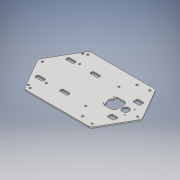
# Autodesk Inventor part: フレームC
Saved by Autodesk Inventor 2017 (Build 210142000, 142)
## iProperties
Created: 2016-08-20
Part Number: フレームC
Material: 一般
Document SubType Name: Modeling
Designer: NN
Density: 1 g/cm^3
Appearance: 既定
Mass: 23.9982 g
Surface Area: 257.222 cm^2
Volume: 23.9982 cm^3
Author: NN
Autodesk Inventor part; units mm, degrees
ref_plane "YZ Plane" through (0, 0, 0) normal (1, 0, 0) x (0, 1, 0)
ref_plane "XZ Plane" through (0, 0, 0) normal (0, 1, 0) x (-1, 0, 0)
ref_plane "XY Plane" through (0, 0, 0) normal (0, 0, 1) x (1, 0, 0)
sketch "スケッチ1" plane through (0, 0, 0) normal (0, 0, 1) x (1, 0, 0)
  line L0 (28.8675, 50) -> (57.735, 0)
  line L1 (57.735, 0) -> (28.8675, -50)
  line L2 (28.8675, -50) -> (-28.8675, -50)
  line L3 (-28.8675, -50) -> (-57.735, 0)
  line L4 (-57.735, 0) -> (-28.8675, 50)
  line L5 (-28.8675, 50) -> (28.8675, 50)
  point P0 (0, 0)
  point P1 (0, 0)
  dimension "d0" = 100
  constraints: 12 end point, 1 coincident, 1 horizontal, 13 other
  measures "d0" distance between parallel lines of L2 L5
extrude "押し出し1" add sketch "スケッチ1" along normal blind 2
sketch "スケッチ2" plane through (0, 0, 2) normal (0, 0, 1) x (1, 0, 0)
  line L0 (57.735, 0) -> (28.8675, 50) projected
  line L1 (28.8675, 50) -> (-28.8675, 50) projected
  line L2 (-28.8675, 50) -> (-57.735, 0) projected
  line L3 (-57.735, 0) -> (-28.8675, -50) projected
  line L4 (-28.8675, -50) -> (28.8675, -50) projected
  line L5 (28.8675, -50) -> (57.735, 0) projected
  line L6 (-50, 86.6025) -> (50, 86.6025)
  line L7 (50, 86.6025) -> (100, 0)
  line L8 (100, 0) -> (50, -86.6025)
  line L9 (50, -86.6025) -> (-50, -86.6025)
  line L10 (-50, -86.6025) -> (-100, 0)
  line L11 (-100, 0) -> (-50, 86.6025)
  line L12 (-28.8675, 50) -> (-71.1325, 50)
  line L13 (-28.8675, -50) -> (-71.1325, -50)
  point P0 (0, 0)
  dimension "d46" = 100
  constraints: 16 end point, 2 point on line, 1 horizontal, 1 parallel, 5 other
  measures "d46" distance of point (0, 0) L10.end
extrude "押し出し2" add sketch "スケッチ2" against normal up to surface (2 mm away) contours L2 L3 L13 L10 L11 L12
fillet "フィレット1" radius 7.5 6 edges at (-100, 0, 1) (-71.1325, -50, 1) (28.8675, -50, 1) (57.735, 0, 1) (28.8675, 50, 1) (-71.1325, 50, 1)
sketch "スケッチ3" plane through (0, 0, 0) normal (0, 0, -1) x (-1, 0, 0)
  arc A0 (73.2976, 46.25) -> (66.8024, 50) centre (66.8024, 42.5) ccw projected
  line L0 (66.8024, 50) -> (-24.5374, 50) projected
  arc A1 (-24.5374, 50) -> (-31.0326, 46.25) centre (-24.5374, 42.5) ccw projected
  line L1 (-31.0326, 46.25) -> (-55.57, 3.75) projected
  arc A2 (-55.57, 3.75) -> (-55.57, -3.75) centre (-49.0748, 0) ccw projected
  line L2 (-55.57, -3.75) -> (-31.0326, -46.25) projected
  arc A3 (-31.0326, -46.25) -> (-24.5374, -50) centre (-24.5374, -42.5) ccw projected
  line L3 (-24.5374, -50) -> (66.8024, -50) projected
  arc A4 (66.8024, -50) -> (73.2976, -46.25) centre (66.8024, -42.5) ccw projected
  line L4 (73.2976, -46.25) -> (97.8349, -3.75) projected
  arc A5 (97.8349, -3.75) -> (97.8349, 3.75) centre (91.3397, 0) ccw projected
  line L5 (97.8349, 3.75) -> (73.2976, 46.25) projected
  point P0 (0, 0)
hole "穴1" at (24.5374, -42.5, 0) at (49.0748, 0, 0) at (24.5374, 42.5, 0) at (-66.8024, 42.5, 0) at (-91.3397, 0, 0) at (-66.8024, -42.5, 0) direction (0, 0, 1) diameter 3 end through all
sketch "スケッチ4" plane through (0, 0, 2) normal (0, 0, 1) x (1, 0, 0)
  line L0 (-60.9252, 24.5) -> (-2.9252, 24.5)
  line L1 (-2.9252, 24.5) -> (-2.9252, -24.5)
  line L2 (-2.9252, -24.5) -> (-60.9252, -24.5)
  line L3 (-60.9252, -24.5) -> (-60.9252, 24.5)
  line L4 (-2.9252, 0) -> (0, 0)
  circle A0 centre (49.0748, 0) radius 1.5 projected
  dimension "d14" = 49
  dimension "d15" = 58
  dimension "d47" = 52
  constraints: 10 end point, 2 parallel, 2 perpendicular, 1 horizontal, 1 midpoint
  measures "d14" distance of L2.end L0.start
  measures "d15" distance of L0.start L0.end
  measures "d47" distance from line of A0.centre L1
hole "穴2" at (-2.9252, 24.5, 2) at (-2.9252, -24.5, 2) at (-60.9252, -24.5, 2) at (-60.9252, 24.5, 2) direction (0, 0, -1) diameter 2.7 end through all
sketch "スケッチ7" plane through (0, 0, 0) normal (0, 0, -1) x (-1, 0, 0)
  circle A0 centre (91.3397, 0) radius 1.5 projected
  line L0 (91.3397, 0) -> (41.7494, 0)
  line L1 (29.9252, -25) -> (41.9252, -25)
  line L2 (41.9252, -25) -> (41.9252, -20)
  line L3 (41.9252, -20) -> (29.9252, -20)
  line L4 (29.9252, -20) -> (29.9252, -25)
  line L5 (29.9252, 25) -> (41.9252, 25)
  line L6 (41.9252, 25) -> (41.9252, 20)
  line L7 (41.9252, 20) -> (29.9252, 20)
  line L8 (29.9252, 20) -> (29.9252, 25)
  circle A1 centre (60.9252, -24.5) radius 1.35 projected
  circle A2 centre (2.9252, 24.5) radius 1.35 projected
  circle A3 centre (2.9252, -24.5) radius 1.35 projected
  circle A4 centre (60.9252, 24.5) radius 1.35 projected
  circle A5 centre (91.3397, 0) radius 1.5 projected
  circle A6 centre (-24.5374, 42.5) radius 1.5 projected
  circle A7 centre (-24.5374, -42.5) radius 1.5 projected
  circle A8 centre (-49.0748, 0) radius 1.5 projected
  circle A9 centre (66.8024, 42.5) radius 1.5 projected
  circle A10 centre (66.8024, -42.5) radius 1.5 projected
  arc A11 (73.2976, 46.25) -> (66.8024, 50) centre (66.8024, 42.5) ccw projected
  line L9 (66.8024, 50) -> (-24.5374, 50) projected
  arc A12 (-24.5374, 50) -> (-31.0326, 46.25) centre (-24.5374, 42.5) ccw projected
  line L10 (-31.0326, 46.25) -> (-55.57, 3.75) projected
  arc A13 (-55.57, 3.75) -> (-55.57, -3.75) centre (-49.0748, 0) ccw projected
  line L11 (-55.57, -3.75) -> (-31.0326, -46.25) projected
  arc A14 (-31.0326, -46.25) -> (-24.5374, -50) centre (-24.5374, -42.5) ccw projected
  line L12 (-24.5374, -50) -> (66.8024, -50) projected
  arc A15 (66.8024, -50) -> (73.2976, -46.25) centre (66.8024, -42.5) ccw projected
  line L13 (73.2976, -46.25) -> (97.8349, -3.75) projected
  arc A16 (97.8349, -3.75) -> (97.8349, 3.75) centre (91.3397, 0) ccw projected
  line L14 (97.8349, 3.75) -> (73.2976, 46.25) projected
  point P0 (0, 0)
  dimension "d35" = 5
  dimension "d36" = 40
  dimension "d37" = 12
  dimension "d75" = 31
  constraints: 18 end point, 4 symmetric about line, 2 horizontal, 2 parallel, 1 perpendicular
  measures "d35" distance between parallel lines of L1 L3
  measures "d36" distance between parallel lines of L7 L3
  measures "d37" distance of L1.start L1.end
  measures "d75" distance from line of A1.centre L4
extrude "押し出し4" cut sketch "スケッチ7" against normal through all contours L4 L3 L2 L1 | L5 L6 L7 L8
fillet "フィレット2" radius 1.5 8 edges at (-41.9252, -25, 1) (-41.9252, -20, 1) (-29.9252, -25, 1) (-29.9252, -20, 1) (-41.9252, 20, 1) (-41.9252, 25, 1) (-29.9252, 20, 1) (-29.9252, 25, 1)
sketch "スケッチ9" plane through (0, 0, 2) normal (0, 0, 1) x (1, 0, 0)
  circle A0 centre (31.2748, 0.0001) radius 2.9 projected
  line L0 (17.0747, -8.7998) -> (17.0748, 8.8002) projected
  arc A1 (17.0748, 8.8002) -> (16.0748, 9.8002) centre (16.0748, 8.8002) ccw projected
  line L1 (16.0748, 9.8002) -> (9.5548, 9.8002) projected
  line L2 (8.5548, 5.1237) -> (8.5548, 8.8002) projected
  arc A2 (9.5548, 9.8002) -> (8.5548, 8.8002) centre (9.5548, 8.8002) ccw projected
  arc A3 (8.5548, 5.1237) -> (8.5547, -5.1233) centre (12.5548, 0.0002) ccw projected
  line L3 (8.5547, -8.7998) -> (8.5547, -5.1233) projected
  arc A4 (8.5547, -8.7998) -> (8.8406, -9.4998) centre (9.5547, -8.7998) ccw projected
  line L4 (16.0747, -9.7998) -> (9.5547, -9.7998) projected
  arc A5 (8.5547, -8.7998) -> (9.5547, -9.7998) centre (9.5547, -8.7998) ccw projected
  arc A6 (16.0747, -9.7998) -> (17.0747, -8.7998) centre (16.0747, -8.7998) ccw projected
  line L5 (17.1748, 8.8002) -> (17.1747, -8.7998)
  arc A7 (16.0747, -9.8998) -> (17.1747, -8.7998) centre (16.0747, -8.7998) ccw
  line L6 (16.0747, -9.8998) -> (9.5547, -9.8998)
  arc A8 (8.4547, -8.7998) -> (9.5547, -9.8998) centre (9.5547, -8.7998) ccw
  line L7 (8.4547, -8.7998) -> (8.4547, -5.1718)
  arc A9 (8.4548, 5.1722) -> (8.4547, -5.1718) centre (12.5548, 0.0002) ccw
  line L8 (8.4548, 5.1722) -> (8.4548, 8.8002)
  arc A10 (9.5548, 9.9002) -> (8.4548, 8.8002) centre (9.5548, 8.8002) ccw
  line L9 (9.5548, 9.9002) -> (16.0748, 9.9002)
  arc A11 (17.1748, 8.8002) -> (16.0748, 9.9002) centre (16.0748, 8.8002) ccw
  circle A12 centre (31.2748, 0.0001) radius 5
  point P0 (0, 0)
  dimension "d48" = 0.1
  dimension "d49" = 10
  constraints: 10 end point, 10 point on circle, 6 centre point, 1 coincident, 9 other
  measures "d48" distance between parallel lines of L5 L0
  measures "d49" diameter of A12
extrude "押し出し6" cut sketch "スケッチ9" against normal through all contours A0 | A6 L4 A5 A4 L3 A3 L2 A2 L1 A1 L0 | L5 A7 L6 A8 L7 A9 L8 A10 L9 A11 | A12
sketch "スケッチ10" plane through (0, 0, 2) normal (0, 0, 1) x (1, 0, 0)
  circle A0 centre (6.3747, -7.6998) radius 0.75 projected
  circle A1 centre (6.3748, 7.7002) radius 0.75 projected
  circle A2 centre (37.4748, 7.2001) radius 0.75 projected
  circle A3 centre (37.4747, -7.1999) radius 0.75 projected
  point P0 (0, 0)
hole "穴4" at (6.3748, 7.7002, 2) at (6.3747, -7.6998, 2) at (37.4748, 7.2001, 2) at (37.4747, -7.1999, 2) direction (0, 0, -1) diameter 1.321 end through all thread size "M1.7x0.35" class "6H" standard "ISO Metric profile"
sketch "スケッチ11" plane through (0, 0, 2) normal (0, 0, 1) x (1, 0, 0)
  arc A0 (8.8407, 9.5002) -> (8.5548, 8.8002) centre (9.5548, 8.8002) ccw projected
  line L0 (8.5547, -8.7998) -> (8.5548, 8.8002) projected
  arc A1 (9.5548, 9.8002) -> (8.5548, 8.8002) centre (9.5548, 8.8002) ccw projected
  line L1 (9.5548, 9.8002) -> (19.2748, 9.8001) projected
  arc A2 (24.2748, 4.8001) -> (19.2748, 9.8001) centre (19.2748, 4.8001) ccw projected
  line L2 (24.2747, -4.7999) -> (24.2748, 4.8001) projected
  arc A3 (19.2747, -9.7999) -> (24.2747, -4.7999) centre (19.2747, -4.7999) ccw projected
  line L3 (9.5547, -9.7998) -> (19.2747, -9.7999) projected
  arc A4 (8.5547, -8.7998) -> (9.5547, -9.7998) centre (9.5547, -8.7998) ccw projected
  arc A5 (24.3748, 4.8001) -> (19.2748, 9.9001) centre (19.2748, 4.8001) ccw
  line L4 (19.2748, 9.9001) -> (9.5548, 9.9002)
  arc A6 (9.5548, 9.9002) -> (8.4548, 8.8002) centre (9.5548, 8.8002) ccw
  line L5 (8.4548, 8.8002) -> (8.4547, -8.7998)
  arc A7 (8.4547, -8.7998) -> (9.5547, -9.8998) centre (9.5547, -8.7998) ccw
  line L6 (9.5547, -9.8998) -> (19.2747, -9.8999)
  arc A8 (19.2747, -9.8999) -> (24.3747, -4.7999) centre (19.2747, -4.7999) ccw
  line L7 (24.3747, -4.7999) -> (24.3748, 4.8001)
  point P0 (0, 0)
  dimension "d59" = 0.1
  constraints: 8 end point, 8 point on circle, 4 centre point, 7 other
  measures "d59" distance between parallel lines of L7 L2
extrude "押し出し7" cut sketch "スケッチ11" against normal through all contours A1 L1 A2 L2 A3 L3 A4 L0 A0 | L7 A8 L6 A7 L5 A6 L4 A5
sketch "スケッチ12" plane through (0, 0, 2) normal (0, 0, 1) x (1, 0, 0)
  line L0 (26.2748, -15.4999) -> (36.2748, -15.4999)
  line L1 (36.2748, -15.4999) -> (36.2748, -22.4999)
  line L2 (36.2748, -22.4999) -> (26.2748, -22.4999)
  line L3 (26.2748, -22.4999) -> (26.2748, -15.4999)
  line L4 (35.0747, -9.7999) -> (16.0747, -9.7998) projected
  arc A0 (-66.8024, 50) -> (-73.2976, 46.25) centre (-66.8024, 42.5) ccw projected
  line L5 (-73.2976, 46.25) -> (-97.8349, 3.75) projected
  arc A1 (-97.8349, 3.75) -> (-97.8349, -3.75) centre (-91.3397, 0) ccw projected
  line L6 (-97.8349, -3.75) -> (-73.2976, -46.25) projected
  arc A2 (-73.2976, -46.25) -> (-66.8024, -50) centre (-66.8024, -42.5) ccw projected
  line L7 (-66.8024, -50) -> (24.5374, -50) projected
  arc A3 (24.5374, -50) -> (31.0326, -46.25) centre (24.5374, -42.5) ccw projected
  line L8 (31.0326, -46.25) -> (55.57, -3.75) projected
  arc A4 (55.57, -3.75) -> (55.57, 3.75) centre (49.0748, 0) ccw projected
  line L9 (55.57, 3.75) -> (31.0326, 46.25) projected
  arc A5 (31.0326, 46.25) -> (24.5374, 50) centre (24.5374, 42.5) ccw projected
  line L10 (24.5374, 50) -> (-66.8024, 50) projected
  circle A6 centre (-66.8024, -42.5) radius 1.5 projected
  circle A7 centre (-66.8024, 42.5) radius 1.5 projected
  circle A8 centre (49.0748, 0) radius 1.5 projected
  circle A9 centre (24.5374, -42.5) radius 1.5 projected
  circle A10 centre (24.5374, 42.5) radius 1.5 projected
  circle A11 centre (-91.3397, 0) radius 1.5 projected
  circle A12 centre (-60.9252, 24.5) radius 1.35 projected
  circle A13 centre (-2.9252, -24.5) radius 1.35 projected
  circle A14 centre (-2.9252, 24.5) radius 1.35 projected
  circle A15 centre (-60.9252, -24.5) radius 1.35 projected
  line L11 (-29.9252, 23.5) -> (-29.9252, 21.5) projected
  arc A16 (-31.4252, 20) -> (-29.9252, 21.5) centre (-31.4252, 21.5) ccw projected
  line L12 (-31.4252, 20) -> (-40.4252, 20) projected
  arc A17 (-41.9252, 21.5) -> (-40.4252, 20) centre (-40.4252, 21.5) ccw projected
  line L13 (-41.9252, 21.5) -> (-41.9252, 23.5) projected
  arc A18 (-40.4252, 25) -> (-41.9252, 23.5) centre (-40.4252, 23.5) ccw projected
  line L14 (-40.4252, 25) -> (-31.4252, 25) projected
  arc A19 (-29.9252, 23.5) -> (-31.4252, 25) centre (-31.4252, 23.5) ccw projected
  line L15 (-41.9252, -23.5) -> (-41.9252, -21.5) projected
  arc A20 (-40.4252, -20) -> (-41.9252, -21.5) centre (-40.4252, -21.5) ccw projected
  line L16 (-40.4252, -20) -> (-31.4252, -20) projected
  arc A21 (-29.9252, -21.5) -> (-31.4252, -20) centre (-31.4252, -21.5) ccw projected
  line L17 (-29.9252, -21.5) -> (-29.9252, -23.5) projected
  arc A22 (-31.4252, -25) -> (-29.9252, -23.5) centre (-31.4252, -23.5) ccw projected
  line L18 (-31.4252, -25) -> (-40.4252, -25) projected
  arc A23 (-41.9252, -23.5) -> (-40.4252, -25) centre (-40.4252, -23.5) ccw projected
  line L19 (9.5548, 9.9002) -> (19.2748, 9.9001) projected
  arc A24 (24.3748, 4.8001) -> (19.2748, 9.9001) centre (19.2748, 4.8001) ccw projected
  line L20 (24.3748, 4.8001) -> (24.3747, -4.7999) projected
  arc A25 (19.2747, -9.8999) -> (24.3747, -4.7999) centre (19.2747, -4.7999) ccw projected
  line L21 (19.2747, -9.8999) -> (9.5547, -9.8998) projected
  arc A26 (8.4547, -8.7998) -> (9.5547, -9.8998) centre (9.5547, -8.7998) ccw projected
  line L22 (8.4547, -8.7998) -> (8.4547, -5.1718) projected
  arc A27 (8.4548, 5.1722) -> (8.4547, -5.1718) centre (12.5548, 0.0002) ccw projected
  line L23 (8.4548, 5.1722) -> (8.4548, 8.8002) projected
  arc A28 (9.5548, 9.9002) -> (8.4548, 8.8002) centre (9.5548, 8.8002) ccw projected
  circle A29 centre (31.2748, 0.0001) radius 5 projected
  circle A30 centre (37.4747, -7.1999) radius 0.6605 projected
  circle A31 centre (6.3747, -7.6998) radius 0.6605 projected
  circle A32 centre (6.3748, 7.7002) radius 0.6605 projected
  circle A33 centre (37.4748, 7.2001) radius 0.6605 projected
  line L24 (31.2748, 0.0001) -> (35.0747, 0.0001)
  line L25 (31.2748, 0.0001) -> (31.2748, -15.4999)
  line L26 (26.2748, 15.5001) -> (36.2748, 15.5001)
  line L27 (36.2748, 15.5001) -> (36.2748, 22.5001)
  line L28 (36.2748, 22.5001) -> (26.2748, 22.5001)
  line L29 (26.2748, 22.5001) -> (26.2748, 15.5001)
  point P0 (0, 0)
  point P1 (35.0747, 9.8001)
  point P2 (31.2748, 15.5001)
  dimension "d62" = 10
  dimension "d63" = 7
  dimension "d64" = 15.5
  constraints: 20 end point, 6 symmetric about line, 2 horizontal, 2 parallel, 2 perpendicular, 1 midpoint
  measures "d62" distance of L1.end L2.end
  measures "d63" distance between parallel lines of L0 L2
  measures "d64" distance between parallel lines of L0 L24
extrude "押し出し8" cut sketch "スケッチ12" against normal through all contours L0 L1 L2 L3 | L29 L28 L27 L26
fillet "フィレット3" radius 1.5 8 edges at (26.2748, 22.5001, 1) (26.2748, 15.5001, 1) (36.2748, 22.5001, 1) (36.2748, 15.5001, 1) (36.2748, -22.4999, 1) (26.2748, -15.4999, 1) (36.2748, -15.4999, 1) (26.2748, -22.4999, 1)
sketch "スケッチ13" plane through (0, 0, 2) normal (0, 0, 1) x (1, 0, 0)
  line L0 (-77.9252, 25) -> (-65.9252, 25)
  line L1 (-65.9252, 25) -> (-65.9252, 20)
  line L2 (-65.9252, 20) -> (-77.9252, 20)
  line L3 (-77.9252, 20) -> (-77.9252, 25)
  line L4 (26.2748, -20.9999) -> (26.2748, -16.9999) projected
  arc A0 (27.7748, -15.4999) -> (26.2748, -16.9999) centre (27.7748, -16.9999) ccw projected
  line L5 (27.7748, -15.4999) -> (34.7748, -15.4999) projected
  arc A1 (36.2748, -16.9999) -> (34.7748, -15.4999) centre (34.7748, -16.9999) ccw projected
  line L6 (36.2748, -16.9999) -> (36.2748, -20.9999) projected
  arc A2 (34.7748, -22.4999) -> (36.2748, -20.9999) centre (34.7748, -20.9999) ccw projected
  line L7 (34.7748, -22.4999) -> (27.7748, -22.4999) projected
  arc A3 (26.2748, -20.9999) -> (27.7748, -22.4999) centre (27.7748, -20.9999) ccw projected
  line L8 (36.2748, 21.0001) -> (36.2748, 17.0001) projected
  arc A4 (34.7748, 15.5001) -> (36.2748, 17.0001) centre (34.7748, 17.0001) ccw projected
  line L9 (34.7748, 15.5001) -> (27.7748, 15.5001) projected
  arc A5 (26.2748, 17.0001) -> (27.7748, 15.5001) centre (27.7748, 17.0001) ccw projected
  line L10 (26.2748, 17.0001) -> (26.2748, 21.0001) projected
  arc A6 (27.7748, 22.5001) -> (26.2748, 21.0001) centre (27.7748, 21.0001) ccw projected
  line L11 (27.7748, 22.5001) -> (34.7748, 22.5001) projected
  arc A7 (36.2748, 21.0001) -> (34.7748, 22.5001) centre (34.7748, 21.0001) ccw projected
  arc A8 (-66.8024, 50) -> (-73.2976, 46.25) centre (-66.8024, 42.5) ccw projected
  line L12 (-73.2976, 46.25) -> (-97.8349, 3.75) projected
  arc A9 (-97.8349, 3.75) -> (-97.8349, -3.75) centre (-91.3397, 0) ccw projected
  line L13 (-97.8349, -3.75) -> (-73.2976, -46.25) projected
  arc A10 (-73.2976, -46.25) -> (-66.8024, -50) centre (-66.8024, -42.5) ccw projected
  line L14 (-66.8024, -50) -> (24.5374, -50) projected
  arc A11 (24.5374, -50) -> (31.0326, -46.25) centre (24.5374, -42.5) ccw projected
  line L15 (31.0326, -46.25) -> (55.57, -3.75) projected
  arc A12 (55.57, -3.75) -> (55.57, 3.75) centre (49.0748, 0) ccw projected
  line L16 (55.57, 3.75) -> (31.0326, 46.25) projected
  arc A13 (31.0326, 46.25) -> (24.5374, 50) centre (24.5374, 42.5) ccw projected
  line L17 (24.5374, 50) -> (-66.8024, 50) projected
  circle A14 centre (-66.8024, -42.5) radius 1.5 projected
  circle A15 centre (-66.8024, 42.5) radius 1.5 projected
  circle A16 centre (49.0748, 0) radius 1.5 projected
  circle A17 centre (24.5374, -42.5) radius 1.5 projected
  circle A18 centre (24.5374, 42.5) radius 1.5 projected
  circle A19 centre (-91.3397, 0) radius 1.5 projected
  circle A20 centre (-60.9252, 24.5) radius 1.35 projected
  circle A21 centre (-2.9252, -24.5) radius 1.35 projected
  circle A22 centre (-2.9252, 24.5) radius 1.35 projected
  circle A23 centre (-60.9252, -24.5) radius 1.35 projected
  line L18 (-29.9252, 23.5) -> (-29.9252, 21.5) projected
  arc A24 (-31.4252, 20) -> (-29.9252, 21.5) centre (-31.4252, 21.5) ccw projected
  line L19 (-31.4252, 20) -> (-40.4252, 20) projected
  arc A25 (-41.9252, 21.5) -> (-40.4252, 20) centre (-40.4252, 21.5) ccw projected
  line L20 (-41.9252, 21.5) -> (-41.9252, 23.5) projected
  arc A26 (-40.4252, 25) -> (-41.9252, 23.5) centre (-40.4252, 23.5) ccw projected
  line L21 (-40.4252, 25) -> (-31.4252, 25) projected
  arc A27 (-29.9252, 23.5) -> (-31.4252, 25) centre (-31.4252, 23.5) ccw projected
  line L22 (-41.9252, -23.5) -> (-41.9252, -21.5) projected
  arc A28 (-40.4252, -20) -> (-41.9252, -21.5) centre (-40.4252, -21.5) ccw projected
  line L23 (-40.4252, -20) -> (-31.4252, -20) projected
  arc A29 (-29.9252, -21.5) -> (-31.4252, -20) centre (-31.4252, -21.5) ccw projected
  line L24 (-29.9252, -21.5) -> (-29.9252, -23.5) projected
  arc A30 (-31.4252, -25) -> (-29.9252, -23.5) centre (-31.4252, -23.5) ccw projected
  line L25 (-31.4252, -25) -> (-40.4252, -25) projected
  arc A31 (-41.9252, -23.5) -> (-40.4252, -25) centre (-40.4252, -23.5) ccw projected
  line L26 (9.5548, 9.9002) -> (19.2748, 9.9001) projected
  arc A32 (24.3748, 4.8001) -> (19.2748, 9.9001) centre (19.2748, 4.8001) ccw projected
  line L27 (24.3748, 4.8001) -> (24.3747, -4.7999) projected
  arc A33 (19.2747, -9.8999) -> (24.3747, -4.7999) centre (19.2747, -4.7999) ccw projected
  line L28 (19.2747, -9.8999) -> (9.5547, -9.8998) projected
  arc A34 (8.4547, -8.7998) -> (9.5547, -9.8998) centre (9.5547, -8.7998) ccw projected
  line L29 (8.4547, -8.7998) -> (8.4547, -5.1718) projected
  arc A35 (8.4548, 5.1722) -> (8.4547, -5.1718) centre (12.5548, 0.0002) ccw projected
  line L30 (8.4548, 5.1722) -> (8.4548, 8.8002) projected
  arc A36 (9.5548, 9.9002) -> (8.4548, 8.8002) centre (9.5548, 8.8002) ccw projected
  circle A37 centre (31.2748, 0.0001) radius 5 projected
  circle A38 centre (37.4747, -7.1999) radius 0.6605 projected
  circle A39 centre (6.3747, -7.6998) radius 0.6605 projected
  circle A40 centre (6.3748, 7.7002) radius 0.6605 projected
  circle A41 centre (37.4748, 7.2001) radius 0.6605 projected
  circle A42 centre (-91.3397, 0) radius 1.5 projected
  line L31 (-91.3397, 0) -> (-81.3975, 0)
  line L32 (-77.9252, -25) -> (-65.9252, -25)
  line L33 (-65.9252, -25) -> (-65.9252, -20)
  line L34 (-65.9252, -20) -> (-77.9252, -20)
  line L35 (-77.9252, -20) -> (-77.9252, -25)
  point P0 (0, 0)
  dimension "d68" = 5
  dimension "d69" = 40
  dimension "d70" = 12
  dimension "d71" = 5
  constraints: 18 end point, 4 symmetric about line, 2 horizontal, 2 parallel, 1 perpendicular
  measures "d68" distance between parallel lines of L0 L2
  measures "d69" distance between parallel lines of L34 L2
  measures "d70" distance of L32.start L32.end
  measures "d71" distance from line of A20.centre L1
extrude "押し出し9" cut sketch "スケッチ13" against normal through all contours L0 L1 L2 L3 | L35 L34 L33 L32
fillet "フィレット4" radius 1.5 8 edges at (-65.9252, -20, 1) (-65.9252, -25, 1) (-77.9252, -25, 1) (-77.9252, -20, 1) (-65.9252, 20, 1) (-65.9252, 25, 1) (-77.9252, 20, 1) (-77.9252, 25, 1)
sketch "スケッチ15" plane through (0, 0, 2) normal (0, 0, 1) x (1, 0, 0)
  line L0 (8.0748, -40) -> (-71.9252, -40)
  line L1 (-71.9252, -40) -> (-71.9252, 40)
  line L2 (-71.9252, 40) -> (8.0748, 40)
  line L3 (8.0748, 40) -> (8.0748, -40)
  line L4 (-77.9252, 21.5) -> (-77.9252, 23.5) projected
  arc A0 (-76.4252, 25) -> (-77.9252, 23.5) centre (-76.4252, 23.5) ccw projected
  line L5 (-76.4252, 25) -> (-67.4252, 25) projected
  arc A1 (-65.9252, 23.5) -> (-67.4252, 25) centre (-67.4252, 23.5) ccw projected
  line L6 (-65.9252, 23.5) -> (-65.9252, 21.5) projected
  arc A2 (-67.4252, 20) -> (-65.9252, 21.5) centre (-67.4252, 21.5) ccw projected
  line L7 (-67.4252, 20) -> (-76.4252, 20) projected
  arc A3 (-77.9252, 21.5) -> (-76.4252, 20) centre (-76.4252, 21.5) ccw projected
  line L8 (-65.9252, -21.5) -> (-65.9252, -23.5) projected
  arc A4 (-67.4252, -25) -> (-65.9252, -23.5) centre (-67.4252, -23.5) ccw projected
  line L9 (-67.4252, -25) -> (-76.4252, -25) projected
  arc A5 (-77.9252, -23.5) -> (-76.4252, -25) centre (-76.4252, -23.5) ccw projected
  line L10 (-77.9252, -23.5) -> (-77.9252, -21.5) projected
  arc A6 (-76.4252, -20) -> (-77.9252, -21.5) centre (-76.4252, -21.5) ccw projected
  line L11 (-76.4252, -20) -> (-67.4252, -20) projected
  arc A7 (-65.9252, -21.5) -> (-67.4252, -20) centre (-67.4252, -21.5) ccw projected
  line L12 (26.2748, -20.9999) -> (26.2748, -16.9999) projected
  arc A8 (27.7748, -15.4999) -> (26.2748, -16.9999) centre (27.7748, -16.9999) ccw projected
  line L13 (27.7748, -15.4999) -> (34.7748, -15.4999) projected
  arc A9 (36.2748, -16.9999) -> (34.7748, -15.4999) centre (34.7748, -16.9999) ccw projected
  line L14 (36.2748, -16.9999) -> (36.2748, -20.9999) projected
  arc A10 (34.7748, -22.4999) -> (36.2748, -20.9999) centre (34.7748, -20.9999) ccw projected
  line L15 (34.7748, -22.4999) -> (27.7748, -22.4999) projected
  arc A11 (26.2748, -20.9999) -> (27.7748, -22.4999) centre (27.7748, -20.9999) ccw projected
  line L16 (36.2748, 21.0001) -> (36.2748, 17.0001) projected
  arc A12 (34.7748, 15.5001) -> (36.2748, 17.0001) centre (34.7748, 17.0001) ccw projected
  line L17 (34.7748, 15.5001) -> (27.7748, 15.5001) projected
  arc A13 (26.2748, 17.0001) -> (27.7748, 15.5001) centre (27.7748, 17.0001) ccw projected
  line L18 (26.2748, 17.0001) -> (26.2748, 21.0001) projected
  arc A14 (27.7748, 22.5001) -> (26.2748, 21.0001) centre (27.7748, 21.0001) ccw projected
  line L19 (27.7748, 22.5001) -> (34.7748, 22.5001) projected
  arc A15 (36.2748, 21.0001) -> (34.7748, 22.5001) centre (34.7748, 21.0001) ccw projected
  arc A16 (-66.8024, 50) -> (-73.2976, 46.25) centre (-66.8024, 42.5) ccw projected
  line L20 (-73.2976, 46.25) -> (-97.8349, 3.75) projected
  arc A17 (-97.8349, 3.75) -> (-97.8349, -3.75) centre (-91.3397, 0) ccw projected
  line L21 (-97.8349, -3.75) -> (-73.2976, -46.25) projected
  arc A18 (-73.2976, -46.25) -> (-66.8024, -50) centre (-66.8024, -42.5) ccw projected
  line L22 (-66.8024, -50) -> (24.5374, -50) projected
  arc A19 (24.5374, -50) -> (31.0326, -46.25) centre (24.5374, -42.5) ccw projected
  line L23 (31.0326, -46.25) -> (55.57, -3.75) projected
  arc A20 (55.57, -3.75) -> (55.57, 3.75) centre (49.0748, 0) ccw projected
  line L24 (55.57, 3.75) -> (31.0326, 46.25) projected
  arc A21 (31.0326, 46.25) -> (24.5374, 50) centre (24.5374, 42.5) ccw projected
  line L25 (24.5374, 50) -> (-66.8024, 50) projected
  circle A22 centre (-66.8024, -42.5) radius 1.5 projected
  circle A23 centre (-66.8024, 42.5) radius 1.5 projected
  circle A24 centre (49.0748, 0) radius 1.5 projected
  circle A25 centre (24.5374, -42.5) radius 1.5 projected
  circle A26 centre (24.5374, 42.5) radius 1.5 projected
  circle A27 centre (-91.3397, 0) radius 1.5 projected
  circle A28 centre (-60.9252, 24.5) radius 1.35 projected
  circle A29 centre (-2.9252, -24.5) radius 1.35 projected
  circle A30 centre (-2.9252, 24.5) radius 1.35 projected
  circle A31 centre (-60.9252, -24.5) radius 1.35 projected
  line L26 (-29.9252, 23.5) -> (-29.9252, 21.5) projected
  arc A32 (-31.4252, 20) -> (-29.9252, 21.5) centre (-31.4252, 21.5) ccw projected
  line L27 (-31.4252, 20) -> (-40.4252, 20) projected
  arc A33 (-41.9252, 21.5) -> (-40.4252, 20) centre (-40.4252, 21.5) ccw projected
  line L28 (-41.9252, 21.5) -> (-41.9252, 23.5) projected
  arc A34 (-40.4252, 25) -> (-41.9252, 23.5) centre (-40.4252, 23.5) ccw projected
  line L29 (-40.4252, 25) -> (-31.4252, 25) projected
  arc A35 (-29.9252, 23.5) -> (-31.4252, 25) centre (-31.4252, 23.5) ccw projected
  line L30 (-41.9252, -23.5) -> (-41.9252, -21.5) projected
  arc A36 (-40.4252, -20) -> (-41.9252, -21.5) centre (-40.4252, -21.5) ccw projected
  line L31 (-40.4252, -20) -> (-31.4252, -20) projected
  arc A37 (-29.9252, -21.5) -> (-31.4252, -20) centre (-31.4252, -21.5) ccw projected
  line L32 (-29.9252, -21.5) -> (-29.9252, -23.5) projected
  arc A38 (-31.4252, -25) -> (-29.9252, -23.5) centre (-31.4252, -23.5) ccw projected
  line L33 (-31.4252, -25) -> (-40.4252, -25) projected
  arc A39 (-41.9252, -23.5) -> (-40.4252, -25) centre (-40.4252, -23.5) ccw projected
  line L34 (9.5548, 9.9002) -> (19.2748, 9.9001) projected
  arc A40 (24.3748, 4.8001) -> (19.2748, 9.9001) centre (19.2748, 4.8001) ccw projected
  line L35 (24.3748, 4.8001) -> (24.3747, -4.7999) projected
  arc A41 (19.2747, -9.8999) -> (24.3747, -4.7999) centre (19.2747, -4.7999) ccw projected
  line L36 (19.2747, -9.8999) -> (9.5547, -9.8998) projected
  arc A42 (8.4547, -8.7998) -> (9.5547, -9.8998) centre (9.5547, -8.7998) ccw projected
  line L37 (8.4547, -8.7998) -> (8.4547, -5.1718) projected
  arc A43 (8.4548, 5.1722) -> (8.4547, -5.1718) centre (12.5548, 0.0002) ccw projected
  line L38 (8.4548, 5.1722) -> (8.4548, 8.8002) projected
  arc A44 (9.5548, 9.9002) -> (8.4548, 8.8002) centre (9.5548, 8.8002) ccw projected
  circle A45 centre (31.2748, 0.0001) radius 5 projected
  circle A46 centre (37.4747, -7.1999) radius 0.6605 projected
  circle A47 centre (6.3747, -7.6998) radius 0.6605 projected
  circle A48 centre (6.3748, 7.7002) radius 0.6605 projected
  circle A49 centre (37.4748, 7.2001) radius 0.6605 projected
  line L39 (-2.9252, -24.5) -> (-60.9252, -24.5)
  circle A50 centre (-60.9252, 24.5) radius 1.35 projected
  line L40 (-2.9252, 24.5) -> (-60.9252, 24.5)
  line L41 (-31.9252, 24.5) -> (-31.9252, -24.5)
  line L42 (-31.9252, 0) -> (-26.2863, 0)
  point P0 (0, 0)
  dimension "d83" = 80
  dimension "d84" = 80
  dimension "d85" = 40
  dimension "d86" = 40
  constraints: 16 end point, 4 horizontal, 3 midpoint, 2 parallel, 1 perpendicular
  measures "d83" distance of L0.end L1.end
  measures "d84" distance of L0.start L0.end
  measures "d85" distance between parallel lines of L42 L0
  measures "d86" distance between parallel lines of L1 L41
hole "穴5" at (-71.9252, -40, 2) at (-71.9252, 40, 2) at (8.0748, 40, 2) at (8.0748, -40, 2) direction (0, 0, -1) diameter 3 end through all
sketch "スケッチ16" plane through (0, 0, 2) normal (0, 0, 1) x (1, 0, 0)
  circle A0 centre (8.0748, 40) radius 1.5 projected
  circle A1 centre (-71.9252, -40) radius 1.5 projected
  circle A2 centre (-71.9252, 40) radius 1.5 projected
  circle A3 centre (8.0748, -40) radius 1.5 projected
  line L0 (-77.9252, 21.5) -> (-77.9252, 23.5) projected
  arc A4 (-76.4252, 25) -> (-77.9252, 23.5) centre (-76.4252, 23.5) ccw projected
  line L1 (-76.4252, 25) -> (-67.4252, 25) projected
  arc A5 (-65.9252, 23.5) -> (-67.4252, 25) centre (-67.4252, 23.5) ccw projected
  line L2 (-65.9252, 23.5) -> (-65.9252, 21.5) projected
  arc A6 (-67.4252, 20) -> (-65.9252, 21.5) centre (-67.4252, 21.5) ccw projected
  line L3 (-67.4252, 20) -> (-76.4252, 20) projected
  arc A7 (-77.9252, 21.5) -> (-76.4252, 20) centre (-76.4252, 21.5) ccw projected
  line L4 (-65.9252, -21.5) -> (-65.9252, -23.5) projected
  arc A8 (-67.4252, -25) -> (-65.9252, -23.5) centre (-67.4252, -23.5) ccw projected
  line L5 (-67.4252, -25) -> (-76.4252, -25) projected
  arc A9 (-77.9252, -23.5) -> (-76.4252, -25) centre (-76.4252, -23.5) ccw projected
  line L6 (-77.9252, -23.5) -> (-77.9252, -21.5) projected
  arc A10 (-76.4252, -20) -> (-77.9252, -21.5) centre (-76.4252, -21.5) ccw projected
  line L7 (-76.4252, -20) -> (-67.4252, -20) projected
  arc A11 (-65.9252, -21.5) -> (-67.4252, -20) centre (-67.4252, -21.5) ccw projected
  line L8 (26.2748, -20.9999) -> (26.2748, -16.9999) projected
  arc A12 (27.7748, -15.4999) -> (26.2748, -16.9999) centre (27.7748, -16.9999) ccw projected
  line L9 (27.7748, -15.4999) -> (34.7748, -15.4999) projected
  arc A13 (36.2748, -16.9999) -> (34.7748, -15.4999) centre (34.7748, -16.9999) ccw projected
  line L10 (36.2748, -16.9999) -> (36.2748, -20.9999) projected
  arc A14 (34.7748, -22.4999) -> (36.2748, -20.9999) centre (34.7748, -20.9999) ccw projected
  line L11 (34.7748, -22.4999) -> (27.7748, -22.4999) projected
  arc A15 (26.2748, -20.9999) -> (27.7748, -22.4999) centre (27.7748, -20.9999) ccw projected
  line L12 (36.2748, 21.0001) -> (36.2748, 17.0001) projected
  arc A16 (34.7748, 15.5001) -> (36.2748, 17.0001) centre (34.7748, 17.0001) ccw projected
  line L13 (34.7748, 15.5001) -> (27.7748, 15.5001) projected
  arc A17 (26.2748, 17.0001) -> (27.7748, 15.5001) centre (27.7748, 17.0001) ccw projected
  line L14 (26.2748, 17.0001) -> (26.2748, 21.0001) projected
  arc A18 (27.7748, 22.5001) -> (26.2748, 21.0001) centre (27.7748, 21.0001) ccw projected
  line L15 (27.7748, 22.5001) -> (34.7748, 22.5001) projected
  arc A19 (36.2748, 21.0001) -> (34.7748, 22.5001) centre (34.7748, 21.0001) ccw projected
  arc A20 (-66.8024, 50) -> (-73.2976, 46.25) centre (-66.8024, 42.5) ccw projected
  line L16 (-73.2976, 46.25) -> (-97.8349, 3.75) projected
  arc A21 (-97.8349, 3.75) -> (-97.8349, -3.75) centre (-91.3397, 0) ccw projected
  line L17 (-97.8349, -3.75) -> (-73.2976, -46.25) projected
  arc A22 (-73.2976, -46.25) -> (-66.8024, -50) centre (-66.8024, -42.5) ccw projected
  line L18 (-66.8024, -50) -> (24.5374, -50) projected
  arc A23 (24.5374, -50) -> (31.0326, -46.25) centre (24.5374, -42.5) ccw projected
  line L19 (31.0326, -46.25) -> (55.57, -3.75) projected
  arc A24 (55.57, -3.75) -> (55.57, 3.75) centre (49.0748, 0) ccw projected
  line L20 (55.57, 3.75) -> (31.0326, 46.25) projected
  arc A25 (31.0326, 46.25) -> (24.5374, 50) centre (24.5374, 42.5) ccw projected
  line L21 (24.5374, 50) -> (-66.8024, 50) projected
  circle A26 centre (-66.8024, -42.5) radius 1.5 projected
  circle A27 centre (-66.8024, 42.5) radius 1.5 projected
  circle A28 centre (49.0748, 0) radius 1.5 projected
  circle A29 centre (24.5374, -42.5) radius 1.5 projected
  circle A30 centre (24.5374, 42.5) radius 1.5 projected
  circle A31 centre (-91.3397, 0) radius 1.5 projected
  circle A32 centre (-60.9252, 24.5) radius 1.35 projected
  circle A33 centre (-2.9252, -24.5) radius 1.35 projected
  circle A34 centre (-2.9252, 24.5) radius 1.35 projected
  circle A35 centre (-60.9252, -24.5) radius 1.35 projected
  line L22 (-29.9252, 23.5) -> (-29.9252, 21.5) projected
  arc A36 (-31.4252, 20) -> (-29.9252, 21.5) centre (-31.4252, 21.5) ccw projected
  line L23 (-31.4252, 20) -> (-40.4252, 20) projected
  arc A37 (-41.9252, 21.5) -> (-40.4252, 20) centre (-40.4252, 21.5) ccw projected
  line L24 (-41.9252, 21.5) -> (-41.9252, 23.5) projected
  arc A38 (-40.4252, 25) -> (-41.9252, 23.5) centre (-40.4252, 23.5) ccw projected
  line L25 (-40.4252, 25) -> (-31.4252, 25) projected
  arc A39 (-29.9252, 23.5) -> (-31.4252, 25) centre (-31.4252, 23.5) ccw projected
  line L26 (-41.9252, -23.5) -> (-41.9252, -21.5) projected
  arc A40 (-40.4252, -20) -> (-41.9252, -21.5) centre (-40.4252, -21.5) ccw projected
  line L27 (-40.4252, -20) -> (-31.4252, -20) projected
  arc A41 (-29.9252, -21.5) -> (-31.4252, -20) centre (-31.4252, -21.5) ccw projected
  line L28 (-29.9252, -21.5) -> (-29.9252, -23.5) projected
  arc A42 (-31.4252, -25) -> (-29.9252, -23.5) centre (-31.4252, -23.5) ccw projected
  line L29 (-31.4252, -25) -> (-40.4252, -25) projected
  arc A43 (-41.9252, -23.5) -> (-40.4252, -25) centre (-40.4252, -23.5) ccw projected
  line L30 (9.5548, 9.9002) -> (19.2748, 9.9001) projected
  arc A44 (24.3748, 4.8001) -> (19.2748, 9.9001) centre (19.2748, 4.8001) ccw projected
  line L31 (24.3748, 4.8001) -> (24.3747, -4.7999) projected
  arc A45 (19.2747, -9.8999) -> (24.3747, -4.7999) centre (19.2747, -4.7999) ccw projected
  line L32 (19.2747, -9.8999) -> (9.5547, -9.8998) projected
  arc A46 (8.4547, -8.7998) -> (9.5547, -9.8998) centre (9.5547, -8.7998) ccw projected
  line L33 (8.4547, -8.7998) -> (8.4547, -5.1718) projected
  arc A47 (8.4548, 5.1722) -> (8.4547, -5.1718) centre (12.5548, 0.0002) ccw projected
  line L34 (8.4548, 5.1722) -> (8.4548, 8.8002) projected
  arc A48 (9.5548, 9.9002) -> (8.4548, 8.8002) centre (9.5548, 8.8002) ccw projected
  circle A49 centre (31.2748, 0.0001) radius 5 projected
  circle A50 centre (37.4747, -7.1999) radius 0.6605 projected
  circle A51 centre (6.3747, -7.6998) radius 0.6605 projected
  circle A52 centre (6.3748, 7.7002) radius 0.6605 projected
  circle A53 centre (37.4748, 7.2001) radius 0.6605 projected
  arc A54 (-66.8024, 48) -> (-71.5655, 45.25) centre (-66.8024, 42.5) ccw
  line L35 (-71.5655, 45.25) -> (-96.1029, 2.75)
  arc A55 (-96.1029, 2.75) -> (-96.1029, -2.75) centre (-91.3397, 0) ccw
  line L36 (-96.1029, -2.75) -> (-71.5655, -45.25)
  arc A56 (-71.5655, -45.25) -> (-66.8024, -48) centre (-66.8024, -42.5) ccw
  line L37 (-66.8024, -48) -> (24.5374, -48)
  arc A57 (24.5374, -48) -> (29.3005, -45.25) centre (24.5374, -42.5) ccw
  line L38 (29.3005, -45.25) -> (53.8379, -2.75)
  arc A58 (53.8379, -2.75) -> (53.8379, 2.75) centre (49.0748, 0) ccw
  line L39 (53.8379, 2.75) -> (29.3005, 45.25)
  arc A59 (29.3005, 45.25) -> (24.5374, 48) centre (24.5374, 42.5) ccw
  line L40 (24.5374, 48) -> (-66.8024, 48)
  point P0 (0, 0)
  dimension "d94" = 2
  constraints: 12 end point, 12 point on circle, 6 centre point, 11 other
  measures "d94" distance between parallel lines of L21 L40
extrude "押し出し11" cut sketch "スケッチ16" against normal through all contours L21 A25 L20 A24 L19 A23 L18 A22 L17 A21 L16 A20
